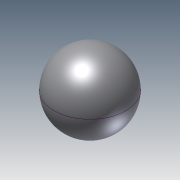
# Autodesk Inventor part: J005234
Saved by Autodesk Inventor 2015 SP1 (Build 190203100, 203)
## iProperties
Created: 2014-08-21
Part Number: J005234
Material: Generic
Vendor: HHMI: JFRC - ID&F
Document SubType Name: Modeling
Designer: arnoldj
Density: 1 g/cm^3
Appearance: Default
Description: MBS BALL
Project: P-201804
RuleStatus: InUse
AfterDocSave0: file://Part Number Cleaner
LAB/DEPT: SVOBODA (LAB)
REQUESTING SCIENTIST: SOFRONIEW, NICK
SURFACE ROUGHNESS: N/A
DESIGN DEPARTMENT: HHMI: JRC - ID&F
SPECIAL FINISH: NONE
ALTERED ITEM PART NUMBER: N/A
ALTERED ITEM VENDOR: N/A
ALTERED ITEM DESCRIPTION: N/A
Author: arnoldj
Revision Number: -
Autodesk Inventor part; units mm, degrees
ref_plane "YZ Plane" through (0, 0, 0) normal (1, 0, 0) x (0, 1, 0)
sketch "Sketch1" plane through (0, 0, 0) normal (0, 0, 1) x (1, 0, 0)
  line L0 (0, 0) -> (0, 116.9406)
  arc A0 (0, 195.2625) -> (0, -195.2625) centre (0, 0) ccw
  line L1 (0, 197.6438) -> (0, 195.2625)
  line L2 (0, -195.2625) -> (0, -197.6438)
  line L3 (-197.7838, 0.0635) -> (-195.326, 0.0635)
  line L4 (-195.326, 0.0635) -> (-195.326, -0.0635)
  line L5 (-195.326, -0.0635) -> (-197.6437, -0.0635)
  line L6 (-286.2656, 0) -> (47.7109, 0) projected
  arc A1 (0, 197.6438) -> (-197.6437, 0.0635) centre (0, 0) ccw
  arc A2 (-197.6437, -0.0635) -> (0, -197.6438) centre (0, 0) ccw
  dimension "d3" = 0.127
  dimension "d4" = 0.0635
  dimension "d5" = 195.326
  constraints: 12 end point, 6 point on circle, 3 centre point, 2 collinear, 2 perpendicular, 1 coincident, 1 horizontal, 1 point on line, 1 vertical
  measures "d3" distance between parallel lines of L3 L5
  measures "d4" distance between parallel lines of L6 L3
  measures "d5" distance from line of L4 A0.centre
revolve "Revolution1" add sketch "Sketch1" angle 360 about axis through (0, 0, 0) along (0, 1, 0)
ref_plane "Work Plane1" through (0, 197.6438, 0) normal (0, 1, 0) x (-1, 0, 0)
ref_plane "Work Plane2" through (0, -197.6438, 0) normal (0, 1, 0) x (-1, 0, 0)
body "Solid1"
